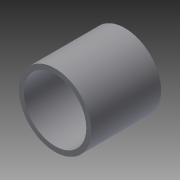
# Autodesk Inventor part: Gearbox Ring Gear 64 to 1
Saved by Autodesk Inventor 2013 (Build 170138000, 138)
## iProperties
Created: 2012-01-14
Part Number: Gearbox Ring Gear 64 to 1
Material: Generic
Document SubType Name: Modeling
Designer: Moses
Density: 1 g/cm^3
Mass: 9.73 g
Surface Area: 82.0866 cm^2
Volume: 9.73 cm^3
Author: Moses
Autodesk Inventor part; units mm, degrees
ref_plane "YZ Plane" through (0, 0, 0) normal (1, 0, 0) x (0, 1, 0)
ref_plane "XZ Plane" through (0, 0, 0) normal (0, 1, 0) x (-1, 0, 0)
ref_plane "XY Plane" through (0, 0, 0) normal (0, 0, 1) x (1, 0, 0)
sketch "Sketch1" plane through (0, 0, 0) normal (0, 0, 1) x (1, 0, 0)
  circle A0 centre (0, 0) radius 18.415
  circle A1 centre (0, 0) radius 15.875
  dimension "d0" = 36.83
  dimension "d1" = 31.75
  constraints: 2 centre point, 2 coincident
  measures "d0" diameter of A0
  measures "d1" diameter of A1
extrude "Extrusion1" add sketch "Sketch1" along normal blind 35.56
body "Solid1"
